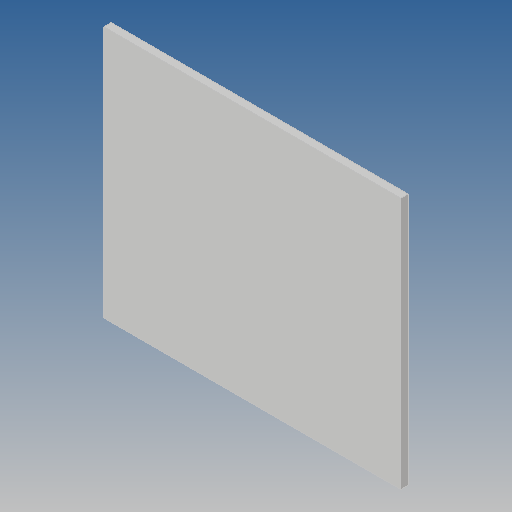
# Autodesk Inventor part: Boden
Saved by Autodesk Inventor 2019 (Build 230136000, 136)
## iProperties
Created: 2022-10-27
Part Number: Boden
Material: Generisch
Document SubType Name: Modeling
Designer: Dominik Schmidt
Density: 1 g/cm^3
Appearance: Vorgabe
Author: Dominik Schmidt
Autodesk Inventor part; units mm, degrees
ref_plane "YZ Plane" through (0, 0, 0) normal (1, 0, 0) x (0, 1, 0)
ref_plane "XZ Plane" through (0, 0, 0) normal (0, 1, 0) x (-1, 0, 0)
ref_plane "XY Plane" through (0, 0, 0) normal (0, 0, 1) x (1, 0, 0)
sketch "Skizze1" plane through (0, 0, 0) normal (0, 0, 1) x (1, 0, 0)
  ellipse E0 centre (-15.2, -12.5548) end of major axis (-12.7, -12.5548) minor radius 2.4737 projected
  ellipse E1 centre (-15.2, -28.3865) end of major axis (-12.7, -28.3865) minor radius 2.4737 projected
  ellipse E2 centre (-15.2, -20.4707) end of major axis (-12.7, -20.4707) minor radius 2.4737 projected
  line L0 (-80.2, -65.9868) -> (-1.2, -65.9868) projected
  line L1 (-1.2, -65.9868) -> (-1.2, 6.2453) projected
  line L2 (-80.2, 6.2453) -> (-80.2, -65.9868) projected
  ellipse E3 centre (-15.2, -53.1236) end of major axis (-18.7, -53.1236) minor radius 3.4632 projected
  ellipse E4 centre (-33.6, -57.5762) end of major axis (-37.6, -57.5762) minor radius 3.9579 (-33.6, -61.5342) -> (-29.6, -57.5762) ccw projected
  line L3 (-33.6, -61.5342) -> (-71.8, -61.5342) projected
  ellipse E5 centre (-71.8, -57.5762) end of major axis (-67.8, -57.5762) minor radius 3.9579 (-75.8, -57.5762) -> (-71.8, -61.5342) ccw projected
  line L4 (-75.8, -57.5762) -> (-75.8, -9.0917) projected
  ellipse E6 centre (-71.8, -9.0917) end of major axis (-67.8, -9.0917) minor radius 3.9579 (-71.8, -5.1337) -> (-75.8, -9.0917) ccw projected
  line L5 (-71.8, -5.1337) -> (-33.6, -5.1337) projected
  ellipse E7 centre (-33.6, -9.0917) end of major axis (-37.6, -9.0917) minor radius 3.9579 (-29.6, -9.0917) -> (-33.6, -5.1337) ccw projected
  line L6 (-29.6, -9.0917) -> (-29.6, -57.5762) projected
  line L7 (0, 0) -> (0, -69.1271) projected
  line L8 (0, -69.1271) -> (-81.4, -69.1271) projected
  line L9 (-81.4, -69.1271) -> (-81.4, 0) projected
  line L10 (-81.4, 0) -> (0, 0) projected
  line L11 (-80.2, -67.9144) -> (-1.2, -67.9144) projected
  line L12 (-1.2, -67.9144) -> (-1.2, -1.2128) projected
  line L13 (-80.2, -1.2128) -> (-80.2, -67.9144) projected
  line L14 (-1.2, -67.9144) -> (-1.2, -1.2128) projected
  line L15 (-80.2, -67.9144) -> (-1.2, -67.9144) projected
  line L16 (-80.2, -1.2128) -> (-80.2, -67.9144) projected
  line L17 (-1.2, -1.2128) -> (-80.2, -1.2128) projected
  line L18 (-81.4, -69.1271) -> (-81.4, 0) projected
  line L19 (0, -69.1271) -> (-81.4, -69.1271) projected
  line L20 (0, 0) -> (0, -69.1271) projected
  line L21 (-81.4, 0) -> (0, 0) projected
  line L22 (-1.2, 6.2453) -> (-80.2, 6.2453) projected
  constraints: 8 other
extrude "Extrusion1" add sketch "Skizze1" along normal blind 2 contours E0 | E1 | E2 | L2 L17 L1 L0 | L13 L11 L12 L1 L10 L7 L8 L9 L2 | L0 L12 L11 L13 | L2 L10 L1 L17 | E3 | L3 E5 L4 E6 L5 E7 L6 E4
